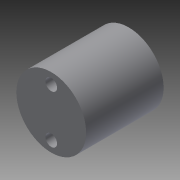
# Autodesk Inventor part: rueda loca
Saved by Autodesk Inventor 2015 (Build 190159000, 159)
## iProperties
Created: 2015-11-29
Part Number: rueda loca
Material: Genérico
Document SubType Name: Modeling
Designer: user
Density: 1 g/cm^3
Appearance: Valor por defecto
Author: user
Autodesk Inventor part; units mm, degrees
ref_plane "YZ Plane" through (0, 0, 0) normal (1, 0, 0) x (0, 1, 0)
ref_plane "XZ Plane" through (0, 0, 0) normal (0, 1, 0) x (-1, 0, 0)
ref_plane "XY Plane" through (0, 0, 0) normal (0, 0, 1) x (1, 0, 0)
sketch "Boceto1" plane through (0, 0, 0) normal (0, 1, 0) x (-1, 0, 0)
  circle A0 centre (0, 0) radius 9
  dimension "d0" = 18
  constraints: 1 centre point, 1 coincident
  measures "d0" diameter of A0
extrude "Extrusión1" add sketch "Boceto1" against normal blind 20
sketch "Boceto3" plane through (0, 0, 0) normal (0, 1, 0) x (1, 0, 0)
  point P0 (0, 0)
sketch "Boceto4" plane through (0, 0, 0) normal (0, 1, 0) x (1, 0, 0)
  circle A0 centre (0, -6.226) radius 1.5
  circle A1 centre (0, 6.226) radius 1.5
  point P0 (0, 0)
  dimension "d6" = 3
  dimension "d7" = 3
  constraints: 2 centre point
  measures "d6" diameter of A0
  measures "d7" diameter of A1
extrude "Extrusión2" cut sketch "Boceto4" against normal blind 20
